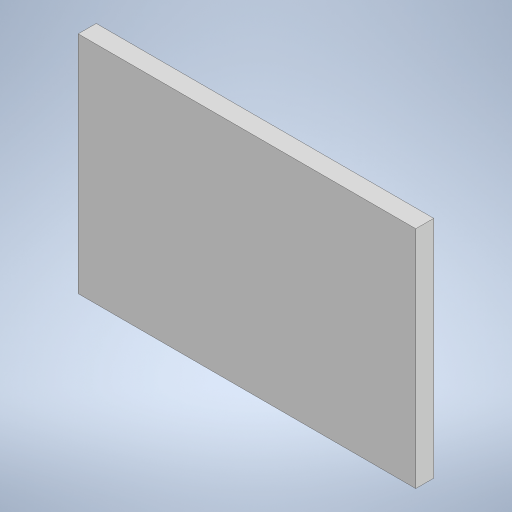
# Autodesk Inventor part: AFSLUITSCHIJF
Saved by Autodesk Inventor 2024 (Build 280153000, 153)
## iProperties
Created: 2024-05-14
Part Number: AFSLUITSCHIJF
Material: Generic
Document SubType Name: Modeling
Designer: Bjarni Heselmans
Density: 1 g/cm^3
Appearance: Default
Author: Bjarni Heselmans
Autodesk Inventor part; units mm, degrees
ref_plane "YZ Plane" through (0, 0, 0) normal (1, 0, 0) x (0, 1, 0)
ref_plane "XZ Plane" through (0, 0, 0) normal (0, 1, 0) x (-1, 0, 0)
ref_plane "XY Plane" through (0, 0, 0) normal (0, 0, 1) x (1, 0, 0)
sketch "Sketch1" plane through (0, 0, 0) normal (0, 0, 1) x (1, 0, 0)
  line L0 (0, 0) -> (-75, 0)
  line L1 (0, 0) -> (75, 0) construction
  line L2 (-75, 0) -> (-75, 4)
  line L3 (-75, 4) -> (0, 4)
  line L4 (0, 4) -> (0, 0)
  dimension "d0" = 75
  dimension "d1" = 180
  dimension "d2" = 4
  constraints: 10 end point, 3 perpendicular, 2 horizontal, 1 collinear
  measures "d0" distance of L0.start L0.end
  measures "d1" angle of L0 L1
  measures "d2" distance of L0.end L2.end
extrude "Extrusion1" add sketch "Sketch1" along normal blind 50
body "Solid1"
